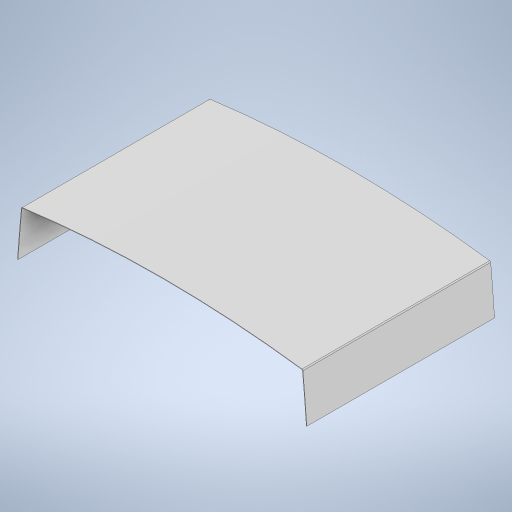
# Autodesk Inventor part: МОО 010 лист спина 1
Saved by Autodesk Inventor 2024.2 (Build 282272000, 272)
## iProperties
Created: 2024-04-18
Part Number: МОО 010 лист спина 1
Material: Stainless Steel AISI 304
Document SubType Name: Sheet Metal
Designer: admin
Density: 8 g/cm^3
Sheet Metal Rule: Default_mm
Sheet Metal Width: 1000,000 mm
Sheet Metal Length: 1999,999 mm
Sheet Metal Area: 1999999,412 mm^2
Appearance: Default
Stock Number: МОО 010 лист спина 1
Flat Pattern Width: 100 cm
Flat Pattern Length: 200 cm
Flat Pattern Area: 20000 cm^2
Author: admin
Autodesk Inventor part; units mm, degrees
ref_plane "YZ Plane" through (0, 0, 0) normal (1, 0, 0) x (0, 1, 0)
ref_plane "XZ Plane" through (0, 0, 0) normal (0, 1, 0) x (-1, 0, 0)
ref_plane "XY Plane" through (0, 0, 0) normal (0, 0, 1) x (1, 0, 0)
sketch "Sketch1" plane through (0, 0, 0) normal (0, 0, 1) x (1, 0, 0)
  line L0 (-750, 0) -> (750, 0) construction
  line L1 (750, 0) -> (750, -2700) construction
  line L2 (750, -2700) -> (-750, -2700) construction
  line L3 (-750, -2700) -> (-750, 0) construction
  line L4 (800, 50) -> (-800, 50) construction
  line L5 (-800, 50) -> (-800, -2750) construction
  line L6 (-800, -2750) -> (800, -2750) construction
  line L7 (800, -2750) -> (800, 50) construction
  line L8 (-850, 100) -> (850, 100) construction
  line L9 (850, 100) -> (850, -2800) construction
  line L10 (850, -2800) -> (-850, -2800) construction
  line L11 (-850, -2800) -> (-850, 100) construction
  arc A0 (750, 0) -> (745.2706, 0.6314) centre (0, -5600) ccw construction
  line L12 (-750, -2100) -> (750, -2100) construction
  arc A1 (-750, 0) -> (-750.4522, -4.7486) centre (10250, -1050) ccw construction
  line L13 (-750, -2100) -> (-111.731, -2698.3772) construction
  line L14 (-107.6273, -2700) -> (107.6273, -2700) construction
  line L15 (111.731, -2698.3772) -> (750, -2100) construction
  arc A2 (750, -2100) -> (771.067, -250.8873) centre (-10250, -1050) ccw construction
  line L16 (-750, 0) -> (-749.6018, -2.9735) construction
  line L17 (750, 0) -> (749.6018, -2.9735) construction
  arc A3 (749.6018, -2.9735) -> (744.8747, -2.3427) centre (0, -5603.0268) ccw construction
  line L18 (-750, 0) -> (-747.0136, -0.2851) construction
  line L19 (750, 0) -> (747.0136, -0.2851) construction
  line L20 (-770.156, -238.4205) -> (-767.1641, -238.6409) construction
  arc A4 (-767.1641, -238.6409) -> (-747.3678, -5.0812) centre (-11767.1672, 811.3268) ccw construction
  line L21 (770.156, -238.4205) -> (767.1641, -238.6409) construction
  arc A5 (767.1641, -238.6409) -> (747.4657, -5.0328) centre (-10252.9895, -1050.2527) ccw construction
  arc A6 (-745.2706, 0.6314) -> (-750.4522, -4.7486) centre (-744.4791, -5.3162) ccw
  arc A7 (750.4522, -4.7486) -> (745.2706, 0.6314) centre (744.4791, -5.3162) ccw
  arc A8 (-744.7715, -2.329) -> (-747.3678, -5.0812) centre (-744.376, -5.3028) ccw construction
  arc A9 (747.4657, -5.0328) -> (744.8747, -2.3427) centre (744.4792, -5.3165) ccw construction
  line L22 (-770.156, -238.4205) -> (-773.1479, -238.2002) construction
  line L23 (-750, -2100) -> (-752.9864, -2100.2851) construction
  arc A10 (-773.1479, -238.2002) -> (-752.9864, -2100.2851) centre (10246.9895, -1050.0326) ccw construction
  line L24 (-750, -2100) -> (-752.0518, -2102.1886) construction
  line L25 (-674.1281, -2171.1299) -> (-676.18, -2173.3185) construction
  line L26 (-752.0518, -2102.1886) -> (-676.18, -2173.3185) construction
  arc A11 (-750.1077, -2098.8714) -> (-749.173, -2100.7753) centre (-747.1212, -2098.5867) ccw construction
  arc A12 (-753.0941, -2099.1563) -> (-751.2249, -2102.9639) centre (-747.1212, -2098.5866) ccw construction
  line L27 (770.156, -238.4205) -> (773.1479, -238.2002) construction
  line L28 (750, -2100) -> (752.9864, -2100.2851) construction
  arc A13 (752.9864, -2100.2851) -> (773.1479, -238.2002) centre (-10246.9895, -1050.0326) ccw construction
  line L29 (674.1281, -2171.1299) -> (676.18, -2173.3185) construction
  line L30 (750, -2100) -> (752.0518, -2102.1886) construction
  line L31 (676.18, -2173.3185) -> (752.0518, -2102.1886) construction
  arc A14 (749.173, -2100.7753) -> (750.1077, -2098.8714) centre (747.1212, -2098.5867) ccw construction
  arc A15 (751.2249, -2102.9639) -> (753.0941, -2099.1563) centre (747.1212, -2098.5866) ccw construction
  line L32 (674.1281, -2171.1299) -> (672.0763, -2168.9413) construction
  line L33 (-674.1281, -2171.1299) -> (-672.0763, -2168.9413) construction
  line L34 (-107.6273, -2697) -> (107.6273, -2697) construction
  line L35 (-672.0763, -2168.9413) -> (-109.6791, -2696.1886) construction
  line L36 (109.6791, -2696.1886) -> (672.0763, -2168.9413) construction
  arc A16 (-111.731, -2698.3772) -> (-107.6273, -2700) centre (-107.6273, -2694) ccw construction
  arc A17 (107.6273, -2700) -> (111.731, -2698.3772) centre (107.6273, -2694) ccw construction
  arc A18 (-109.6791, -2696.1886) -> (-107.6273, -2697) centre (-107.6273, -2694) ccw construction
  arc A19 (107.6273, -2697) -> (109.6791, -2696.1886) centre (107.6273, -2694) ccw construction
  line L37 (-672.0763, -2168.9413) -> (-681.1955, -2160.392) construction
  line L38 (-681.1955, -2160.392) -> (-683.2473, -2162.5806) construction
  line L39 (-676.18, -2173.3185) -> (-667.0607, -2181.8678) construction
  line L40 (-667.0607, -2181.8678) -> (-665.0089, -2179.6791) construction
  line L41 (672.0763, -2168.9413) -> (681.1955, -2160.392) construction
  line L42 (681.1955, -2160.392) -> (683.2473, -2162.5806) construction
  line L43 (676.18, -2173.3185) -> (667.0607, -2181.8678) construction
  line L44 (667.0607, -2181.8678) -> (665.0089, -2179.6791) construction
  arc A20 (-747.3678, -5.0812) -> (-747.0136, -0.2851) centre (-11767.1672, 811.3268) ccw construction
  arc A21 (-744.7715, -2.329) -> (-749.6018, -2.9735) centre (0, -5603.0268) ccw construction
  arc A22 (744.8747, -2.3427) -> (-744.7715, -2.329) centre (0, -5603.0268) ccw construction
  arc A23 (747.4657, -5.0328) -> (747.0136, -0.2851) centre (-10252.9895, -1050.2527) ccw construction
  arc A24 (-770.156, -238.4205) -> (-771.067, -250.8873) centre (10250, -1050) ccw
  arc A25 (770.156, -238.4205) -> (769.2309, -225.9548) centre (-10250, -1050) ccw
  line L45 (-769.2309, -225.9548) -> (-772.2225, -225.7311) construction
  line L46 (-771.067, -250.8873) -> (-768.0749, -251.1042) construction
  arc A26 (-772.2225, -225.7311) -> (-773.1479, -238.2002) centre (10247.0082, -1049.778) ccw construction
  arc A27 (-767.1641, -238.6409) -> (-768.0749, -251.1042) centre (10252.992, -1050.2186) ccw construction
  arc A28 (-771.067, -250.8873) -> (-750, -2100) centre (10250, -1050) ccw construction
  arc A29 (-769.2309, -225.9548) -> (-770.156, -238.4205) centre (10250, -1050) ccw
  arc A30 (-750.4522, -4.7486) -> (-769.2309, -225.9548) centre (10250, -1050) ccw
  arc A31 (-745.2706, 0.6314) -> (-750, 0) centre (0, -5600) ccw construction
  arc A32 (745.2706, 0.6314) -> (-745.2706, 0.6314) centre (0, -5600) ccw
  arc A33 (750.4522, -4.7486) -> (750, 0) centre (-10250, -1050) ccw construction
  line L47 (771.067, -250.8873) -> (768.0749, -251.1042) construction
  line L48 (769.2309, -225.9548) -> (772.2225, -225.7311) construction
  arc A34 (768.0749, -251.1042) -> (767.1641, -238.6409) centre (-10252.992, -1050.2186) ccw construction
  arc A35 (773.1479, -238.2002) -> (772.2225, -225.7311) centre (-10247.0082, -1049.778) ccw construction
  arc A36 (769.2309, -225.9548) -> (750.4522, -4.7486) centre (-10250, -1050) ccw
  arc A37 (771.067, -250.8873) -> (770.156, -238.4205) centre (-10250, -1050) ccw
  point P0 (0, 0)
  point P1 (0, 0)
  point P2 (-110, -2700)
  point P3 (110, -2700)
  dimension "d54" = 1500
  dimension "d55" = 2700
  dimension "d56" = 50
  dimension "d57" = 50
  dimension "d58" = 2100
  dimension "d59" = 220
  dimension "d60" = 3
  dimension "d61" = 239.271
  dimension "d63" = 3
  dimension "d64" = 239.271
  dimension "d66" = 6
  dimension "d68" = 6
  dimension "d69" = 3
  dimension "d70" = 3
  dimension "d71" = 104
  dimension "d72" = 3
  dimension "d73" = 6
  dimension "d74" = 104
  dimension "d75" = 3
  dimension "d77" = 6
  dimension "d81" = 3
  dimension "d82" = 6
  dimension "d83" = 6
  dimension "d84" = 3
  dimension "d86" = 3
  dimension "d91" = 12.5
  dimension "d92" = 12.5
  dimension "d93" = 12.5
  dimension "d94" = 12.5
  dimension "d101" = 12.5
  dimension "d102" = 12.5
  dimension "d103" = 12.5
  dimension "d104" = 12.5
  measures "d54" distance of L0.start L0.end
  measures "d55" distance of L0.end L1.end
  measures "d56" distance between parallel lines of L0 L4
  measures "d57" distance between parallel lines of L4 L8
  measures "d58" distance between parallel lines of L12 L0
  measures "d59" distance of point (-110, -2700) point (110, -2700)
  measures "d60" distance of L0.start L16.end
  measures "d61" distance of L20.start L0.start
  measures "d63" distance of L0.start L18.end
  measures "d64" distance of L21.start L0.end
  measures "d66" radius of A6
  measures "d68" radius of A7
  measures "d69" radius of A8
  measures "d70" radius of A9
  measures "d71" distance of L25.start L12.start
  measures "d72" radius of A11
  measures "d73" radius of A12
  measures "d74" distance of L29.start L12.end
  measures "d75" radius of A14
  measures "d77" radius of A15
  measures "d81" distance between parallel lines of L2 L34
  measures "d82" radius of A16
  measures "d83" radius of A17
  measures "d84" radius of A18
  measures "d86" radius of A19
  measures "d91" distance of L33.end L37.end
  measures "d92" distance of L25.end L39.end
  measures "d93" distance of L32.end L41.end
  measures "d94" distance of L29.end L43.end
  measures "d101" distance of L45.start L20.start
  measures "d102" distance of L46.start L20.start
  measures "d103" distance of L21.start L48.start
  measures "d104" distance of L47.start L21.start
contour flange "Contour Flange2" sketch "Sketch1" thickness 3 bend radius 3 width 1000 along (0, 0, 1) mid plane no both sides no wall seen from (770.6133, -244.6538, 0) lies toward (-0.9973406, -0.072882, 0) curves A37 A25 A36 A7 A32 A6 A30 A29 A24
bend "Bend2"
corner "Corner2"
equation "\"d36\" = Thickness"
equation "\"d37\" = BendReliefWidth"
equation "\"d38\" = BendReliefDepth"
equation "\"d39\" = MinimumRemnant"
equation "\"d40\" = TransitionRadius"
equation "\"d42\" = BendRadius"
equation "\"d44\" = CornerReliefSize"
equation "\"d45\" = GapSize"
equation "\"d46\" = JacobiRadiusSize"
equation "\"BendRadius\" = Thickness"
equation "\"BendReliefWidth\" = Thickness"
equation "\"BendReliefDepth\" = 0.5 * Thickness"
equation "\"CornerReliefSize\" = 4 * Thickness"
equation "\"MinimumRemnant\" = 2 * Thickness"
equation "\"TransitionRadius\" = BendRadius"
equation "\"JacobiRadiusSize\" = BendRadius"
equation "\"GapSize\" = Thickness"
equation "\"Thickness\" = 3"
body "Solid3"
